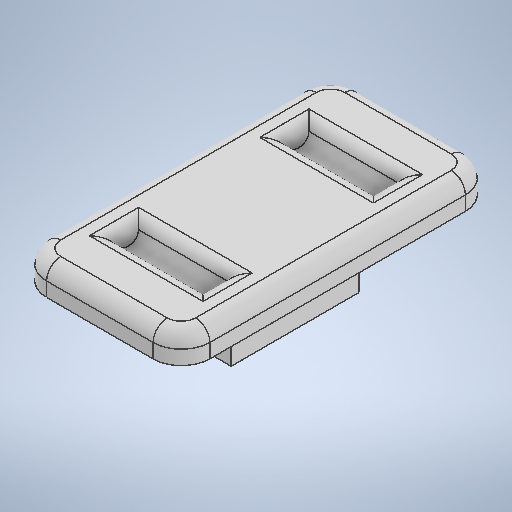
# Autodesk Inventor part: Power Switch
Saved by Autodesk Inventor 2025 (Build 290162000, 162)
## iProperties
Created: 2025-12-15
Part Number: Power Switch
Material: Generic
Document SubType Name: Modeling
Designer: User
Density: 1 g/cm^3
Appearance: Default
Author: User
Autodesk Inventor part; units mm, degrees
ref_plane "YZ Plane" through (0, 0, 0) normal (1, 0, 0) x (0, 1, 0)
ref_plane "XZ Plane" through (0, 0, 0) normal (0, 1, 0) x (-1, 0, 0)
ref_plane "XY Plane" through (0, 0, 0) normal (0, 0, 1) x (1, 0, 0)
sketch "Sketch1" plane through (0, 0, 0) normal (0, 1, 0) x (-1, 0, 0)
  line L0 (0, 0) -> (2.75, 0)
  line L1 (2.75, 0) -> (2.75, -4.5)
  line L2 (2.75, -4.5) -> (0, -4.5)
  line L3 (0, -4.5) -> (0, 0)
  dimension "d0" = 2.75
  dimension "d1" = 4.5
  constraints: 8 end point, 2 parallel, 1 horizontal, 1 perpendicular
  measures "d0" distance of L1.end L2.end
  measures "d1" distance of L0.end L1.end
extrude "Extrusion1" add sketch "Sketch1" along normal blind 2.1
sketch "Sketch2" plane through (0, 2.1, 0) normal (0, 1, 0) x (1, 0, 0)
  line L0 (-4.25, -3.25) -> (1.5, -3.25)
  line L1 (1.5, -3.25) -> (1.5, 7.75)
  line L2 (1.5, 7.75) -> (-4.25, 7.75)
  line L3 (-4.25, 7.75) -> (-4.25, -3.25)
  line L4 (0, 4.5) -> (-2.75, 4.5) projected
  line L5 (-2.75, 4.5) -> (-2.75, 0) projected
  line L6 (-2.75, 0) -> (0, 0) projected
  line L7 (0, 0) -> (0, 4.5) projected
  point P0 (-1.375, -3.25)
  point P1 (-1.375, 0)
  point P2 (-4.25, 2.25)
  point P3 (-2.75, 2.25)
  point P4 (1.5, 2.25)
  dimension "d4" = 1.5
  dimension "d5" = 11
  constraints: 8 end point, 5 midpoint, 2 parallel, 1 horizontal, 1 horizontal alignment, 1 perpendicular, 1 vertical alignment
  measures "d4" distance from line of point (1.5, 2.25) L7
  measures "d5" distance of L2.end L0.start
extrude "Extrusion2" add sketch "Sketch2" along normal blind 1 contours L3 L2 L1 L0 | L7 L6 L5 L4
sketch "Sketch3" plane through (0, 0, 0) normal (0, -1, 0) x (1, 0, 0)
  line L0 (0, -4.5) -> (-2.75, -4.5) construction
  line L1 (-2.75, -4.5) -> (0, 0) construction
  line L2 (0, 0) -> (-2.75, 0) construction
  line L3 (0, 0) -> (0, -4.5) construction
  line L4 (-2.75, 0) -> (0, -4.5) construction
  line L5 (-0.875, -1.575) -> (-1.875, -1.575)
  line L6 (-1.875, -2.925) -> (-0.875, -1.575) construction
  line L7 (-1.875, -2.925) -> (-1.075, -2.925)
  line L8 (-0.875, -1.575) -> (-1.875, -1.575)
  line L9 (-1.875, -1.575) -> (-1.875, -2.925)
  line L10 (-1.875, -2.925) -> (-0.875, -2.925)
  line L11 (-0.875, -2.925) -> (-0.875, -1.575)
  line L12 (-0.875, -1.575) -> (-1.875, -2.925) construction
  line L13 (-1.875, -1.575) -> (-0.875, -2.925) construction
  point P0 (-1.375, -2.25)
  dimension "d22" = 1
  dimension "d23" = 1.35
  constraints: 24 end point, 4 midpoint, 4 parallel, 2 horizontal, 1 perpendicular
  measures "d22" distance between parallel lines of L9 L11
  measures "d23" distance between parallel lines of L10 L5
extrude "Extrusion3" cut sketch "Sketch3" against normal blind 1.5
fillet "Fillet1" radius 1 8 edges at (-2.75, 2.1, -2.25) (-1.375, 2.1, -4.5) (0, 2.1, -2.25) (-1.375, 2.1, 0) (-4.25, 2.6, -7.75) (-4.25, 2.6, 3.25) (1.5, 2.6, -7.75) (1.5, 2.6, 3.25)
fillet "Fillet2" radius 0.5 8 edges at (1.2071, 3.1, 2.9571) (1.5, 3.1, -2.25) (1.2071, 3.1, -7.4571) (-1.375, 3.1, -7.75) (-3.9571, 3.1, -7.4571) (-4.25, 3.1, -2.25) (-3.9571, 3.1, 2.9571) (-1.375, 3.1, 3.25)
sketch "Sketch4" plane through (0, 3.1, 0) normal (0, 1, 0) x (1, 0, 0)
  line L0 (-2.875, -1.25) -> (0.125, -1.25)
  line L1 (0.125, -1.25) -> (0.125, -0.25)
  line L2 (0.125, -0.25) -> (-2.875, -0.25)
  line L3 (-2.875, -0.25) -> (-2.875, -1.25)
  line L4 (-2.875, -1.25) -> (0.125, -0.25) construction
  line L5 (0.125, -1.25) -> (-2.875, -0.25) construction
  line L6 (0.125, 5.75) -> (-2.875, 5.75)
  line L7 (-2.875, 5.75) -> (-2.875, 4.75)
  line L8 (-2.875, 4.75) -> (0.125, 4.75)
  line L9 (0.125, 4.75) -> (0.125, 5.75)
  line L10 (0.125, 5.75) -> (-2.875, 4.75) construction
  line L11 (-2.875, 5.75) -> (0.125, 4.75) construction
  line L12 (0.5, -2.75) -> (-3.25, -2.75) projected
  line L13 (-3.25, 7.25) -> (0.5, 7.25) projected
  point P0 (0, 0)
  point P1 (-1.375, -0.75)
  point P2 (-1.375, 5.25)
  point P3 (-1.375, -2.75)
  dimension "d15" = 3
  dimension "d16" = 1
  dimension "d17" = 2
  dimension "d18" = 2
  constraints: 24 end point, 5 midpoint, 4 parallel, 2 equal length, 2 horizontal, 2 perpendicular, 2 vertical alignment
  measures "d15" distance of L0.start L0.end
  measures "d16" distance between parallel lines of L2 L0
  measures "d17" distance from line of L12 point (-1.375, -0.75)
  measures "d18" distance from line of L13 point (-1.375, 5.25)
extrude "Extrusion4" cut sketch "Sketch4" against normal blind 0.5
fillet "Fillet3" radius 0.5 12 edges at (-2.875, 3.1, 0.75) (-1.375, 3.1, 0.25) (0.125, 3.1, 0.75) (-1.375, 3.1, 1.25) (-1.375, 3.1, -4.75) (-2.875, 3.1, -5.25) (-1.375, 3.1, -5.75) (0.125, 3.1, -5.25) (-1.375, 2.6, -5.75) (-1.375, 2.6, -4.75) (-1.375, 2.6, 1.25) (-1.375, 2.6, 0.25)
equation "\"d18\" = d17"
body "Solid1"
